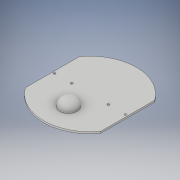
# Autodesk Inventor part: Base Plate
Saved by Autodesk Inventor 2019 (Build 230136000, 136)
## iProperties
Created: 2019-10-19
Part Number: Base Plate
Material: Generic
Document SubType Name: Modeling
Designer: Bryce V
Density: 1 g/cm^3
Appearance: Default
Author: Bryce V
## iProperties of the stored document Base Plate_3DPrint.ipt
Created: 2019-10-19
Part Number: Base Plate_3DPrint
Material: Generic
Document SubType Name: Modeling
Designer: Bryce V
Density: 1 g/cm^3
Appearance: Default
Author: Bryce V
Autodesk Inventor part; units mm, degrees
ref_plane "YZ Plane" through (0, 0, 0) normal (1, 0, 0) x (0, 1, 0)
ref_plane "XZ Plane" through (0, 0, 0) normal (0, 1, 0) x (-1, 0, 0)
ref_plane "XY Plane" through (0, 0, 0) normal (0, 0, 1) x (1, 0, 0)
sketch "Sketch1" plane through (0, 0, 0) normal (0, 1, 0) x (-1, 0, 0)
  line L0 (44.45, 31.7246) -> (44.45, -31.7246)
  line L1 (-44.45, -31.7246) -> (-44.45, 31.7246)
  arc A0 (-44.45, -31.7246) -> (44.45, -31.7246) centre (0, 0) ccw
  arc A1 (44.45, 31.7246) -> (-44.45, 31.7246) centre (0, 0) ccw
  line L2 (44.45, 0) -> (41.91, 0)
  circle A2 centre (41.91, 0) radius 1.27
  line L3 (41.91, 0) -> (21.59, 0)
  circle A3 centre (21.59, 0) radius 1.27
  line L4 (0, -54.61) -> (0, 54.61)
  circle A4 centre (-41.91, 0) radius 1.27
  circle A5 centre (-21.59, 0) radius 1.27
  dimension "d3" = 88.9
  dimension "d4" = 2.54
  dimension "d5" = 2.54
  dimension "d6" = 20.32
  dimension "d7" = 2.54
  constraints: 10 end point, 6 centre point, 6 point on circle, 3 coincident, 2 horizontal, 2 symmetric about line, 1 midpoint, 2 other
  measures "d3" distance between parallel lines of L1 L0
  measures "d4" distance of L2.start L2.end
  measures "d5" diameter of A2
  measures "d6" distance of L3.start L3.end
  measures "d7" diameter of A3
extrude "Extrusion1" add sketch "Sketch1" along normal blind 2.032
sketch "Sketch2" plane through (0, 2.032, 0) normal (0, 1, 0) x (1, 0, 0)
  circle A0 centre (0, -25.3797) radius 10.16
  point P0 (0, 0)
  dimension "d10" = 20.32
  constraints: 1 centre point
  measures "d10" diameter of A0
extrude "Extrusion2" add sketch "Sketch2" along normal blind 10.16
fillet "Fillet1" radius 10.16 1 edges at (-10.16, 12.192, 25.3797)
body "Solid1"
